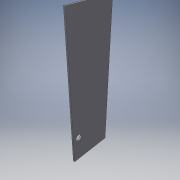
# Autodesk Inventor part: back board (for assembly)
Saved by Autodesk Inventor 2016 (Build 200138000, 138)
## iProperties
Created: 2017-10-23
Part Number: back board (for assembly)
Material: Generic
Document SubType Name: Modeling
Designer: student
Density: 1 g/cm^3
Appearance: Default
Author: student
Autodesk Inventor part; units mm, degrees
ref_plane "YZ Plane" through (0, 0, 0) normal (1, 0, 0) x (0, 1, 0)
ref_plane "XZ Plane" through (0, 0, 0) normal (0, 1, 0) x (-1, 0, 0)
ref_plane "XY Plane" through (0, 0, 0) normal (0, 0, 1) x (1, 0, 0)
sketch "Sketch1" plane through (0, 0, 0) normal (1, 0, 0) x (0, 1, 0)
  line L0 (-787.4, -234.95) -> (787.4, -234.95)
  line L1 (787.4, -234.95) -> (787.4, 234.95)
  line L2 (787.4, 234.95) -> (-787.4, 234.95)
  line L3 (-787.4, 234.95) -> (-787.4, -234.95)
  line L4 (-787.4, -234.95) -> (787.4, 234.95) construction
  line L5 (787.4, -234.95) -> (-787.4, 234.95) construction
  point P0 (0, 0)
  dimension "d0" = 1574.8
  dimension "d1" = 469.9
  constraints: 12 end point, 2 midpoint, 2 parallel, 1 horizontal, 1 perpendicular
  measures "d0" distance of L1.end L2.end
  measures "d1" distance of L0.end L1.end
extrude "Extrusion1" add sketch "Sketch1" along normal blind 19.05
sketch "Sketch2" plane through (0, 0, 0) normal (-1, 0, 0) x (0, 0, 1)
  circle A0 centre (163.83, -482.6) radius 38.1
  line L0 (234.95, 787.4) -> (234.95, -787.4) projected
  line L1 (234.95, -787.4) -> (-234.95, -787.4) projected
  point P0 (0, 0)
  point P1 (0, 0)
  dimension "d5" = 76.2
  dimension "d8" = 71.12
  dimension "d9" = 304.8
  constraints: 1 centre point
  measures "d5" diameter of A0
  measures "d8" distance from line of A0.centre L0
  measures "d9" distance from line of L1 A0.centre
extrude "Extrusion2" cut sketch "Sketch2" against normal blind 25.4
body "Solid1"
